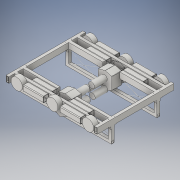
# Autodesk Inventor part: BaseSuperstructure
Saved by Autodesk Inventor 2016 (Build 200138000, 138)
## iProperties
Created: 2018-01-19
Part Number: BaseSuperstructure
Material: Generic
Document SubType Name: Modeling
Designer: New User
Density: 1 g/cm^3
Appearance: Polycarbonate - Clear
Author: New User
Autodesk Inventor part; units mm, degrees
ref_plane "YZ Plane" through (0, 0, 0) normal (1, 0, 0) x (0, 1, 0)
ref_plane "XZ Plane" through (0, 0, 0) normal (0, 1, 0) x (-1, 0, 0)
ref_plane "XY Plane" through (0, 0, 0) normal (0, 0, 1) x (1, 0, 0)
sketch "Sketch1" plane through (0, 0, 0) normal (0, 1, 0) x (-1, 0, 0)
  line L0 (0, -685.8) -> (0, 0)
  line L1 (25.4, -50.8) -> (689.3542, -50.8)
  line L2 (787.4, -76.2) -> (25.4, -76.2)
  line L3 (787.4, -635) -> (25.4, -635)
  line L4 (787.4, -609.6) -> (25.4, -609.6)
  line L5 (787.4, -127) -> (482.6, -127)
  line L6 (482.6, -127) -> (482.6, -152.4)
  line L7 (482.6, -533.4) -> (482.6, -558.8)
  line L8 (482.6, -558.8) -> (787.4, -558.8)
  line L9 (25.4, -558.8) -> (330.2, -558.8)
  line L10 (330.2, -558.8) -> (330.2, -533.4)
  line L11 (330.2, -533.4) -> (25.4, -533.4)
  line L12 (25.4, -152.4) -> (330.2, -152.4)
  line L13 (330.2, -127) -> (25.4, -127)
  line L14 (330.2, -127) -> (330.2, -152.4)
  line L15 (0, 0) -> (25.4, 0)
  line L16 (787.4, 0) -> (812.8, 0)
  line L17 (787.4, -76.2) -> (787.4, -127)
  line L18 (787.4, -558.8) -> (787.4, -609.6)
  line L19 (787.4, -635) -> (787.4, -685.8)
  line L20 (812.8, -685.8) -> (787.4, -685.8)
  line L21 (25.4, -685.8) -> (0, -685.8)
  line L22 (25.4, -635) -> (25.4, -685.8)
  line L23 (25.4, -558.8) -> (25.4, -609.6)
  line L24 (25.4, -152.4) -> (25.4, -533.4)
  line L25 (25.4, 0) -> (25.4, -50.8)
  line L26 (25.4, -76.2) -> (25.4, -127)
  line L27 (689.3542, -50.8) -> (787.4, -50.8)
  line L28 (787.4, -50.8) -> (787.4, 0)
  line L29 (812.8, 0) -> (812.8, -152.4)
  line L30 (812.8, -539.9129) -> (812.8, -685.8)
  line L31 (482.6, -152.4) -> (482.6, -152.4)
  line L32 (508, -152.4) -> (787.3559, -152.4)
  line L33 (660.3559, -533.4) -> (508, -533.4)
  line L34 (482.6, -533.4) -> (482.6, -533.4)
  line L35 (660.3559, -533.4) -> (787.3559, -533.4)
  line L36 (787.3559, -152.4) -> (787.4, -152.4)
  line L37 (787.3559, -533.4) -> (787.4, -533.4)
  line L38 (482.6, -152.4) -> (508, -152.4)
  line L39 (482.6, -533.4) -> (508, -533.4)
  line L40 (787.3559, -152.4) -> (787.3559, -533.4)
  line L41 (812.8, -539.9129) -> (812.8, -152.4)
  dimension "d0" = 685.8
  dimension "d1" = 812.8
  dimension "d4" = 25.4
  dimension "d5" = 25.4
  dimension "d8" = 50.8
  dimension "d9" = 25.4
  dimension "d10" = 50.8
  dimension "d42" = 304.8
  dimension "d43" = 25.4
  dimension "d44" = 25.4
  dimension "d45" = 25.4
  dimension "d46" = 25.4
  dimension "d101" = 50.8
  dimension "d102" = 50.8
  dimension "d103" = 25.4
  dimension "d104" = 50.8
  dimension "d105" = 25.4
  dimension "d108" = 50.8
  dimension "d117" = 50.8
  dimension "d134" = 304.8
  dimension "d135" = 304.8
  dimension "d136" = 25.4
  dimension "d137" = 25.4
  constraints: 84 end point, 63 perpendicular, 8 horizontal, 8 parallel, 6 point on line, 3 equal length
  measures "d0" distance of L16.end L20.start
  measures "d1" distance of L20.start L0.start
  measures "d4" distance between parallel lines of L3 L4
  measures "d5" distance between parallel lines of L2 L1
  measures "d8" distance between parallel lines of L4 L9
  measures "d9" distance of L9.end L10.end
  measures "d10" distance between parallel lines of L2 L5
  measures "d42" distance between parallel lines of L10 L23
  measures "d43" distance between parallel lines of L23 L0
  measures "d44" distance between parallel lines of L0 L24
  measures "d45" distance between parallel lines of L0 L26
  measures "d46" distance between parallel lines of L0 L25
  measures "d101" distance of L15.end L1.start
  measures "d102" distance between parallel lines of L2 L13
  measures "d103" distance between parallel lines of L5 L32
  measures "d104" distance of L3.start L19.end
  measures "d105" distance between parallel lines of L33 L8
  measures "d108" distance of L3.end L21.start
  measures "d117" distance of L27.end L16.start
  measures "d134" distance of L7.end L8.end
  measures "d135" distance of L5.start L5.end
  measures "d136" distance between parallel lines of L29 L17
  measures "d137" distance between parallel lines of L30 L18
extrude "Frame" add sketch "Sketch1" along normal blind 50.8
sketch "Sketch4" plane through (-25.4, 0, -76.2) normal (-1, 0, 0) x (0, 0, 1)
  line L0 (-50.8, 50.8) -> (0, 50.8) projected
  line L1 (0, 0) -> (-50.8, 0) projected
  line L2 (-6.35, 50.8) -> (-44.45, 50.8)
  line L3 (-50.8, 44.45) -> (-50.8, 6.35)
  line L4 (-44.45, 0) -> (-6.35, 0)
  line L5 (0, 6.35) -> (0, 44.45)
  arc A0 (-44.45, 50.8) -> (-50.8, 44.45) centre (-44.45, 44.45) ccw
  arc A1 (-50.8, 6.35) -> (-44.45, 0) centre (-44.45, 6.35) ccw
  arc A2 (0, 44.45) -> (-6.35, 50.8) centre (-6.35, 44.45) ccw
  arc A3 (-6.35, 0) -> (0, 6.35) centre (-6.35, 6.35) ccw
  line L6 (-533.4, 50.8) -> (-482.6, 50.8) projected
  line L7 (-482.6, 0) -> (-482.6, 50.8) projected
  line L8 (-527.05, 50.8) -> (-488.95, 50.8)
  line L9 (-482.6, 44.45) -> (-482.6, 6.35)
  line L10 (-488.95, 0) -> (-527.05, 0)
  line L11 (-533.4, 6.35) -> (-533.4, 44.45)
  arc A4 (-482.6, 44.45) -> (-488.95, 50.8) centre (-488.95, 44.45) ccw
  arc A5 (-533.4, 6.35) -> (-527.05, 0) centre (-527.05, 6.35) ccw
  arc A6 (-527.05, 50.8) -> (-533.4, 44.45) centre (-527.05, 44.45) ccw
  arc A7 (-488.95, 0) -> (-482.6, 6.35) centre (-488.95, 6.35) ccw
  line L12 (-527.05, 3.175) -> (-488.95, 3.175)
  arc A8 (-488.95, 3.175) -> (-485.775, 6.35) centre (-488.95, 6.35) ccw
  line L13 (-485.775, 6.35) -> (-485.775, 44.45)
  arc A9 (-485.775, 44.45) -> (-488.95, 47.625) centre (-488.95, 44.45) ccw
  line L14 (-488.95, 47.625) -> (-527.05, 47.625)
  arc A10 (-527.05, 47.625) -> (-530.225, 44.45) centre (-527.05, 44.45) ccw
  line L15 (-530.225, 44.45) -> (-530.225, 6.35)
  arc A11 (-530.225, 6.35) -> (-527.05, 3.175) centre (-527.05, 6.35) ccw
  line L16 (-6.35, 3.175) -> (-44.45, 3.175)
  arc A12 (-47.625, 6.35) -> (-44.45, 3.175) centre (-44.45, 6.35) ccw
  line L17 (-47.625, 6.35) -> (-47.625, 44.45)
  arc A13 (-44.45, 47.625) -> (-47.625, 44.45) centre (-44.45, 44.45) ccw
  line L18 (-44.45, 47.625) -> (-6.35, 47.625)
  arc A14 (-3.175, 44.45) -> (-6.35, 47.625) centre (-6.35, 44.45) ccw
  line L19 (-3.175, 44.45) -> (-3.175, 6.35)
  arc A15 (-6.35, 3.175) -> (-3.175, 6.35) centre (-6.35, 6.35) ccw
  line L20 (76.2, 0) -> (76.2, 50.8) projected
  line L21 (31.75, 50.8) -> (69.85, 50.8)
  line L22 (76.2, 44.45) -> (76.2, 6.35)
  line L23 (69.85, 0) -> (31.75, 0)
  line L24 (25.4, 6.35) -> (25.4, 44.45)
  line L25 (25.4, 50.8) -> (76.2, 0) construction
  line L26 (76.2, 50.8) -> (25.4, 0) construction
  arc A16 (69.85, 0) -> (76.2, 6.35) centre (69.85, 6.35) ccw
  arc A17 (76.2, 44.45) -> (69.85, 50.8) centre (69.85, 44.45) ccw
  arc A18 (31.75, 50.8) -> (25.4, 44.45) centre (31.75, 44.45) ccw
  arc A19 (25.4, 6.35) -> (31.75, 0) centre (31.75, 6.35) ccw
  line L27 (-565.15, 50.8) -> (-603.25, 50.8)
  line L28 (-609.6, 44.45) -> (-609.6, 6.35)
  line L29 (-603.25, 0) -> (-565.15, 0)
  line L30 (-558.8, 6.35) -> (-558.8, 44.45)
  line L31 (-558.8, 50.8) -> (-609.6, 0) construction
  line L32 (-609.6, 50.8) -> (-558.8, 0) construction
  arc A20 (-565.15, 0) -> (-558.8, 6.35) centre (-565.15, 6.35) ccw
  arc A21 (-558.8, 44.45) -> (-565.15, 50.8) centre (-565.15, 44.45) ccw
  arc A22 (-603.25, 50.8) -> (-609.6, 44.45) centre (-603.25, 44.45) ccw
  arc A23 (-609.6, 6.35) -> (-603.25, 0) centre (-603.25, 6.35) ccw
  line L33 (-565.15, 3.175) -> (-603.25, 3.175)
  arc A24 (-606.425, 6.35) -> (-603.25, 3.175) centre (-603.25, 6.35) ccw
  line L34 (-606.425, 6.35) -> (-606.425, 44.45)
  arc A25 (-603.25, 47.625) -> (-606.425, 44.45) centre (-603.25, 44.45) ccw
  line L35 (-603.25, 47.625) -> (-565.15, 47.625)
  arc A26 (-561.975, 44.45) -> (-565.15, 47.625) centre (-565.15, 44.45) ccw
  line L36 (-561.975, 44.45) -> (-561.975, 6.35)
  arc A27 (-565.15, 3.175) -> (-561.975, 6.35) centre (-565.15, 6.35) ccw
  line L37 (73.025, 6.35) -> (73.025, 44.45)
  arc A28 (73.025, 44.45) -> (69.85, 47.625) centre (69.85, 44.45) ccw
  line L38 (69.85, 47.625) -> (31.75, 47.625)
  arc A29 (31.75, 47.625) -> (28.575, 44.45) centre (31.75, 44.45) ccw
  line L39 (28.575, 44.45) -> (28.575, 6.35)
  arc A30 (28.575, 6.35) -> (31.75, 3.175) centre (31.75, 6.35) ccw
  line L40 (31.75, 3.175) -> (69.85, 3.175)
  arc A31 (69.85, 3.175) -> (73.025, 6.35) centre (69.85, 6.35) ccw
  point P0 (50.8, 25.4)
  point P1 (-584.2, 25.4)
  dimension "d24" = 6.35
  dimension "d25" = 6.35
  dimension "d106" = 6.35
  dimension "d109" = 6.35
  constraints: 72 end point, 64 point on circle, 32 centre point, 32 tangent, 24 point on line, 16 parallel, 12 equal radius, 8 perpendicular, 4 horizontal, 4 midpoint, 28 other
  measures "d24" radius of A0
  measures "d25" radius of A4
  measures "d106" radius of A16
  measures "d109" radius of A20
extrude "tubes" add sketch "Sketch4" along normal blind 774.7 contours L0 A2 L5 A3 L1 A1 L3 A0 | L6 A4 L7 A7 L10 A5 L11 A6 | A16 L23 A19 L24 A18 L21 A17 L20 | A21 L30 A20 L29 A23 L28 A22 L27
sketch "Sketch17" plane through (0, 0, 0) normal (0, -1, 0) x (1, 0, 0)
  line L0 (-25.4, 0) -> (-152.4, 0)
  line L1 (-152.4, 0) -> (-152.4, -50.8)
  line L2 (-152.4, -50.8) -> (-25.4, -50.8)
  line L3 (-25.4, -50.8) -> (-25.4, 0)
  line L4 (-152.4, -69.6871) -> (-25.4, -69.6871)
  line L5 (-25.4, -69.6871) -> (-25.4, -127)
  line L6 (-25.4, -127) -> (-152.4, -127)
  line L7 (-152.4, -127) -> (-152.4, -69.6871)
  line L8 (-25.4, -558.8) -> (-25.4, -565.15) projected
  line L9 (-25.4, -558.8) -> (-152.4, -558.8)
  line L10 (-152.4, -558.8) -> (-152.4, -609.6)
  line L11 (-152.4, -609.6) -> (-25.4, -609.6)
  line L12 (-25.4, -609.6) -> (-25.4, -558.8)
  line L13 (-25.4, -685.8) -> (-152.4, -685.8)
  line L14 (-152.4, -685.8) -> (-152.4, -638.175)
  line L15 (-152.4, -638.175) -> (-25.4, -638.175)
  line L16 (-25.4, -638.175) -> (-25.4, -685.8)
  line L17 (-787.4, 0) -> (-787.4, -6.35) projected
  line L18 (-787.4, 0) -> (-660.4, 0)
  line L19 (-660.4, 0) -> (-660.4, -50.8)
  line L20 (-660.4, -50.8) -> (-787.4, -50.8)
  line L21 (-787.4, -50.8) -> (-787.4, 0)
  line L22 (-787.4, -76.2) -> (-660.4, -76.2)
  line L23 (-660.4, -76.2) -> (-660.4, -127)
  line L24 (-660.4, -127) -> (-787.4, -127)
  line L25 (-787.4, -127) -> (-787.4, -76.2)
  line L26 (-787.4, -558.8) -> (-787.4, -565.15) projected
  line L27 (-787.4, -558.8) -> (-660.4, -558.8)
  line L28 (-660.4, -558.8) -> (-660.4, -609.6)
  line L29 (-660.4, -609.6) -> (-787.4, -609.6)
  line L30 (-787.4, -609.6) -> (-787.4, -558.8)
  line L31 (-787.4, -635) -> (-660.4, -635)
  line L32 (-660.4, -635) -> (-660.4, -685.8)
  line L33 (-660.4, -685.8) -> (-787.4, -685.8)
  line L34 (-787.4, -685.8) -> (-787.4, -635)
  line L35 (-330.2, 0) -> (-482.6, 0)
  line L36 (-482.6, 0) -> (-482.6, -50.8)
  line L37 (-482.6, -50.8) -> (-330.2, -50.8)
  line L38 (-330.2, -50.8) -> (-330.2, 0)
  line L39 (-330.2, -76.2) -> (-482.6, -76.2)
  line L40 (-482.6, -76.2) -> (-482.6, -127)
  line L41 (-482.6, -127) -> (-330.2, -127)
  line L42 (-330.2, -127) -> (-330.2, -76.2)
  line L43 (-482.6, -558.8) -> (-330.2, -558.8)
  line L44 (-330.2, -558.8) -> (-330.2, -609.6)
  line L45 (-330.2, -609.6) -> (-482.6, -609.6)
  line L46 (-482.6, -609.6) -> (-482.6, -558.8)
  line L47 (-330.2, -635) -> (-482.6, -635)
  line L48 (-482.6, -635) -> (-482.6, -685.8)
  line L49 (-482.6, -685.8) -> (-330.2, -685.8)
  line L50 (-330.2, -685.8) -> (-330.2, -635)
  dimension "d116" = 127
  dimension "d118" = 127
  dimension "d119" = 177.8
  dimension "d120" = 177.8
  dimension "d127" = 177.8
  dimension "d128" = 177.8
  dimension "d130" = 177.8
  dimension "d131" = 177.8
  dimension "d133" = 127
  constraints: 96 end point, 24 parallel, 12 horizontal, 12 perpendicular, 7 point on line
  measures "d116" distance of L0.start L0.end
  measures "d118" distance of L17.start L18.end
  measures "d119" distance between parallel lines of L38 L1
  measures "d120" distance between parallel lines of L19 L36
  measures "d127" distance between parallel lines of L42 L7
  measures "d128" distance between parallel lines of L23 L40
  measures "d130" distance between parallel lines of L14 L50
  measures "d131" distance between parallel lines of L32 L48
  measures "d133" distance of L5.end L6.end
extrude "Extrusion19" cut sketch "Sketch17" against normal blind 50.8
sketch "Sketch19" plane through (-787.4, 50.8, -609.6) normal (0, 0, 1) x (1, 0, 0)
  line L0 (-25.4, -50.8) -> (-25.4, 0) projected
  line L1 (319.0875, -15.875) -> (381, 0)
  line L2 (381, 0) -> (441.325, -15.875)
  line L3 (441.325, -15.875) -> (441.325, -124.4763)
  line L4 (441.325, -124.4763) -> (381, -155.575)
  line L5 (381, -155.575) -> (319.0875, -124.4763)
  line L6 (319.0875, -124.4763) -> (319.0875, -15.875)
  point P0 (787.4, -50.8)
  constraints: 12 end point, 1 parallel
extrude "Extrusion20" add sketch "Sketch19" along normal blind 131.572
sketch "Sketch23" plane through (-787.4, 0, -76.2) normal (0, 0, -1) x (-1, 0, 0)
  line L0 (-319.0875, -73.6763) -> (-381, -104.775) projected
  line L1 (-381, -104.775) -> (-319.0875, -73.6763)
  line L2 (-319.0875, 34.925) -> (-319.0875, -73.6763) projected
  line L3 (-319.0875, -73.6763) -> (-319.0875, 34.925)
  line L4 (-319.0875, 34.925) -> (-381, 50.8)
  line L5 (-441.325, -73.6763) -> (-441.325, 34.925) projected
  line L6 (-441.325, 34.925) -> (-441.325, -73.6763)
  line L7 (-441.325, -73.6763) -> (-381, -104.775)
  line L8 (-441.325, 34.925) -> (-381, 50.8)
  point P0 (-787.4, 0)
  constraints: 12 end point, 2 collinear, 1 vertical
extrude "Extrusion25" add sketch "Sketch23" along normal blind 131.572
sketch "Sketch25" plane through (-787.4, 0, -207.772) normal (0, 0, -1) x (-1, 0, 0)
  circle A0 centre (-380.3805, -90.287) radius 25.4
  circle A1 centre (-337.9892, -53.4748) radius 25.4
  circle A2 centre (-374.3738, -8.7689) radius 25.4
  point P0 (-787.4, 0)
  dimension "d170" = 50.8
  dimension "d171" = 50.8
  dimension "d172" = 50.8
  constraints: 3 centre point
  measures "d170" diameter of A0
  measures "d171" diameter of A1
  measures "d172" diameter of A2
extrude "Extrusion26" add sketch "Sketch25" along normal blind 114.3
sketch "Sketch26" plane through (-787.4, 50.8, -478.028) normal (0, 0, 1) x (1, 0, 0)
  arc A0 (355.0213, -142.5259) -> (405.7206, -142.831) centre (380.3805, -141.087) ccw projected
  circle A1 centre (380.3805, -141.087) radius 25.4
  circle A2 centre (337.9892, -104.2748) radius 25.4 projected
  circle A3 centre (337.9892, -104.2748) radius 25.4
  circle A4 centre (374.3738, -59.5689) radius 25.4 projected
  circle A5 centre (374.3738, -59.5689) radius 25.4
  point P0 (787.4, -50.8)
  point P1 (347.5192, -134.6478)
  point P2 (354.3407, -128.3917)
  constraints: 3 centre point, 3 coincident, 1 other
extrude "Extrusion27" add sketch "Sketch26" along normal blind 114.3
sketch "Sketch22" plane through (-25.4, 0.8507, -638.175) normal (0, 0, -1) x (-1, 0, 0)
  circle A0 centre (63.5, 24.5493) radius 50.8
  circle A1 centre (381, 24.5493) radius 50.8
  circle A2 centre (698.5, 24.5493) radius 50.8
  line L0 (0, -0.8507) -> (0, 49.9493) projected
  line L1 (762, -0.8507) -> (762, 49.9493) projected
  point P0 (-25.4, -0.8507)
  dimension "d154" = 101.6
  dimension "d155" = 63.5
  dimension "d156" = 381
  dimension "d157" = 63.5
  constraints: 3 centre point, 2 equal radius
  measures "d154" diameter of A2
  measures "d155" distance from line of L0 A0.centre
  measures "d156" distance from line of L0 A1.centre
  measures "d157" distance from line of L1 A2.centre
extrude "Wheels" add sketch "Sketch22" along normal blind 44.45
sketch "Sketch18" plane through (-787.4, 50.8, -50.8) normal (0, 0, 1) x (1, 0, 0)
  circle A0 centre (698.5, -25.4) radius 50.8
  circle A1 centre (63.5, -25.4) radius 50.8
  circle A2 centre (381, -25.4) radius 50.8
  line L0 (762, -50.8) -> (762, 0) projected
  line L1 (127, -6.35) -> (127, -44.45) projected
  point P0 (787.4, -50.8)
  dimension "d123" = 101.6
  dimension "d124" = 63.5
  dimension "d125" = 63.5
  dimension "d126" = 381
  constraints: 3 centre point, 2 equal radius
  measures "d123" diameter of A0
  measures "d124" distance from line of L0 A0.centre
  measures "d125" distance from line of L1 A1.centre
  measures "d126" distance from line of L0 A2.centre
extrude "Wheels2" add sketch "Sketch18" along normal blind 44.45
sketch "Sketch27" plane through (-468.3125, -73.6763, -76.2) normal (-1, 0, 0) x (0, 0, 1)
  line L0 (-527.05, -50.8) -> (-488.95, -50.8)
  line L1 (-488.95, -50.8) -> (-488.95, 149.225)
  line L2 (-488.95, 149.225) -> (-527.05, 149.225)
  line L3 (-527.05, 149.225) -> (-527.05, -50.8)
  line L4 (-44.45, -14.2875) -> (-44.45, 125.4125)
  line L5 (-44.45, 125.4125) -> (-6.35, 125.4125)
  line L6 (-6.35, 125.4125) -> (-6.35, -14.2875)
  line L7 (-6.35, -14.2875) -> (-6.35, -79.375)
  line L8 (-6.35, -79.375) -> (-44.45, -79.375)
  line L9 (-44.45, -79.375) -> (-44.45, -14.2875)
  point P0 (76.2, 73.6763)
  constraints: 20 end point, 3 parallel, 3 perpendicular, 1 horizontal, 1 vertical
extrude "Extrusion29" cut sketch "Sketch27" against normal blind 127
sketch "Sketch28" plane through (-468.3125, -73.6763, -82.55) normal (0, 0, -1) x (-1, 0, 0)
  line L0 (-115.8875, 4.7625) -> (-114.0873, 11.0555)
  line L1 (-114.0873, 11.0555) -> (-107.7373, 12.643)
  line L2 (-107.7373, 12.643) -> (-103.1875, 7.9375)
  line L3 (-103.1875, 7.9375) -> (-104.9877, 1.6445)
  line L4 (-104.9877, 1.6445) -> (-111.3377, 0.057)
  line L5 (-111.3377, 0.057) -> (-115.8875, 4.7625)
  line L6 (-68.2625, -20.6375) -> (-65.0875, -15.1382)
  line L7 (-65.0875, -15.1382) -> (-58.7375, -15.1382)
  line L8 (-58.7375, -15.1382) -> (-55.5625, -20.6375)
  line L9 (-55.5625, -20.6375) -> (-58.7375, -26.1368)
  line L10 (-58.7375, -26.1368) -> (-65.0875, -26.1368)
  line L11 (-65.0875, -26.1368) -> (-68.2625, -20.6375)
  line L12 (-17.9184, 4.7625) -> (-14.7434, 10.2618)
  line L13 (-14.7434, 10.2618) -> (-8.3934, 10.2618)
  line L14 (-8.3934, 10.2618) -> (-5.2184, 4.7625)
  line L15 (-5.2184, 4.7625) -> (-8.3934, -0.7368)
  line L16 (-8.3934, -0.7368) -> (-14.7434, -0.7368)
  line L17 (-14.7434, -0.7368) -> (-17.9184, 4.7625)
  line L18 (-105.9066, 95.25) -> (-111.9358, 92.4597)
  line L19 (-111.9358, 92.4597) -> (-117.3669, 96.2859)
  line L20 (-117.3669, 96.2859) -> (-116.7688, 102.9025)
  line L21 (-116.7688, 102.9025) -> (-110.7396, 105.6928)
  line L22 (-110.7396, 105.6928) -> (-105.3085, 101.8666)
  line L23 (-105.3085, 101.8666) -> (-105.9066, 95.25)
  line L24 (-17.9184, 98.5583) -> (-14.5168, 104.4501)
  line L25 (-14.5168, 104.4501) -> (-7.7135, 104.4501)
  line L26 (-7.7135, 104.4501) -> (-4.3119, 98.5583)
  line L27 (-4.3119, 98.5583) -> (-7.7135, 92.6665)
  line L28 (-7.7135, 92.6665) -> (-14.5168, 92.6665)
  line L29 (-14.5168, 92.6665) -> (-17.9184, 98.5583)
  point P0 (-468.3125, 73.6763)
  point P1 (-109.5375, 6.35)
  point P2 (-61.9125, -20.6375)
  point P3 (-11.5684, 4.7625)
  point P4 (-111.3377, 99.0763)
  point P5 (-11.1151, 98.5583)
  constraints: 60 end point, 65 other
extrude "Extrusion30" add sketch "Sketch28" along normal blind 65.0875
sketch "Sketch29" plane through (-468.3125, -73.6763, -565.15) normal (0, 0, -1) x (-1, 0, 0)
  line L0 (-68.2625, -20.6375) -> (-65.0875, -15.1382)
  line L1 (-65.0875, -15.1382) -> (-58.7375, -15.1382)
  line L2 (-58.7375, -15.1382) -> (-55.5625, -20.6375)
  line L3 (-55.5625, -20.6375) -> (-58.7375, -26.1368)
  line L4 (-58.7375, -26.1368) -> (-65.0875, -26.1368)
  line L5 (-65.0875, -26.1368) -> (-68.2625, -20.6375)
  line L6 (-111.125, 0) -> (-116.2712, 4.8042)
  line L7 (-116.2712, 4.8042) -> (-114.6837, 11.663)
  line L8 (-114.6837, 11.663) -> (-107.95, 13.7176)
  line L9 (-107.95, 13.7176) -> (-102.8038, 8.9134)
  line L10 (-102.8038, 8.9134) -> (-104.3913, 2.0546)
  line L11 (-104.3913, 2.0546) -> (-111.125, 0)
  line L12 (-112.7125, 106.3625) -> (-109.6472, 110.092)
  line L13 (-109.6472, 110.092) -> (-104.8847, 109.3022)
  line L14 (-104.8847, 109.3022) -> (-103.1875, 104.7828)
  line L15 (-103.1875, 104.7828) -> (-106.2528, 101.0533)
  line L16 (-106.2528, 101.0533) -> (-111.0153, 101.8431)
  line L17 (-111.0153, 101.8431) -> (-112.7125, 106.3625)
  line L18 (-16.2587, 2.0546) -> (-16.2587, 8.9134)
  line L19 (-16.2587, 8.9134) -> (-10.3188, 12.3428)
  line L20 (-10.3188, 12.3428) -> (-4.3788, 8.9134)
  line L21 (-4.3788, 8.9134) -> (-4.3788, 2.0546)
  line L22 (-4.3788, 2.0546) -> (-10.3188, -1.3748)
  line L23 (-10.3188, -1.3748) -> (-16.2587, 2.0546)
  arc A0 (-17.9184, 73.6763) -> (-17.9184, 124.4763) centre (-61.9125, 99.0763) ccw projected
  line L24 (-7.7135, 93.1867) -> (-14.0662, 92.9266)
  line L25 (-14.0662, 92.9266) -> (-17.4679, 98.2982)
  line L26 (-17.4679, 98.2982) -> (-14.5168, 103.9299)
  line L27 (-14.5168, 103.9299) -> (-8.164, 104.19)
  line L28 (-8.164, 104.19) -> (-4.7624, 98.8184)
  line L29 (-4.7624, 98.8184) -> (-7.7135, 93.1867)
  point P0 (-468.3125, 73.6763)
  point P1 (-61.9125, -20.6375)
  point P2 (-109.5375, 6.8588)
  point P3 (-107.95, 105.5727)
  point P4 (-10.3188, 5.484)
  point P5 (-11.1151, 98.5583)
  constraints: 60 end point, 1 point on circle, 1 point on line, 65 other
extrude "Extrusion31" add sketch "Sketch29" along normal blind 41.275
fillet "Fillet1" radius 3.175 11 edges at (-346.075, 34.925, -521.589) (-406.4, 50.8, -521.589) (-468.3125, 34.925, -521.589) (-468.3125, 34.925, -164.211) (-346.075, 34.925, -164.211) (-346.075, -73.6763, -164.211) (-406.4, -104.775, -164.211) (-468.3125, -73.6763, -164.211) (-406.4, -104.775, -521.589) (-346.075, -73.6763, -521.589) (-468.3125, -73.6763, -521.589)
sketch "Sketch30" plane through (0, 0, -685.8) normal (0, 0, -1) x (-1, 0, 0)
  line L0 (809.625, 3.175) -> (790.575, 3.175)
  line L1 (790.575, 3.175) -> (790.575, 47.625)
  line L2 (790.575, 47.625) -> (809.625, 47.625)
  line L3 (809.625, 47.625) -> (809.625, 3.175)
  line L4 (812.8, 0) -> (812.8, 50.8) projected
  line L5 (787.4, 0) -> (812.8, 0) projected
  line L6 (787.4, 0) -> (787.4, 50.8) projected
  line L7 (787.4, 50.8) -> (812.8, 50.8) projected
  line L8 (22.225, 3.175) -> (3.175, 3.175)
  line L9 (3.175, 3.175) -> (3.175, 47.625)
  line L10 (3.175, 47.625) -> (22.225, 47.625)
  line L11 (22.225, 47.625) -> (22.225, 3.175)
  line L12 (0, 0) -> (0, 50.8) projected
  dimension "d189" = 3.175
  dimension "d190" = 3.175
  dimension "d191" = 3.175
  dimension "d192" = 3.175
  constraints: 16 end point, 4 parallel, 2 horizontal, 2 perpendicular
  measures "d189" distance between parallel lines of L4 L3
  measures "d190" distance between parallel lines of L5 L0
  measures "d191" distance between parallel lines of L6 L1
  measures "d192" distance between parallel lines of L7 L2
extrude "Extrusion32" cut sketch "Sketch30" against normal blind 685.8 contours L0 L1 L2 L3 | L8 L9 L10 L11
sketch "Sketch33" plane through (0, 0, 0) normal (0, -1, 0) x (1, 0, 0)
  line L0 (0, 0) -> (0, -685.8) projected
  line L1 (-25.4, -152.4) -> (0, -152.4)
  line L2 (0, -152.4) -> (0, -127)
  line L3 (0, -127) -> (-25.4, -127)
  line L4 (-25.4, -127) -> (-25.4, -152.4)
  line L5 (-330.2, -533.4) -> (-25.4, -533.4) projected
  line L6 (-25.4, -533.4) -> (0, -533.4)
  line L7 (0, -533.4) -> (0, -558.8)
  line L8 (0, -558.8) -> (-25.4, -558.8)
  line L9 (-25.4, -558.8) -> (-25.4, -533.4)
  line L10 (-482.6, -127) -> (-787.4, -127) projected
  line L11 (-787.4, -127) -> (-812.8, -127)
  line L12 (-812.8, -127) -> (-812.8, -152.4)
  line L13 (-812.8, -152.4) -> (-787.4, -152.4)
  line L14 (-787.4, -152.4) -> (-787.4, -127)
  line L15 (-482.6, -558.8) -> (-787.4, -558.8) projected
  line L16 (-787.4, -558.8) -> (-812.8, -558.8)
  line L17 (-812.8, -558.8) -> (-812.8, -533.4)
  line L18 (-812.8, -533.4) -> (-787.4, -533.4)
  line L19 (-787.4, -533.4) -> (-787.4, -558.8)
  point P0 (-533.4, -127)
  constraints: 32 end point, 8 parallel, 5 point on line, 4 horizontal, 4 perpendicular
extrude "Extrusion35" add sketch "Sketch33" along normal blind 114.3
sketch "Sketch34" plane through (-812.8, 0, 0) normal (-1, 0, 0) x (0, 0, 1)
  line L0 (-152.4, -114.3) -> (-127, -114.3) projected
  line L1 (-127, -114.3) -> (-152.4, -114.3)
  line L2 (-152.4, -114.3) -> (-152.4, -139.7)
  line L3 (-152.4, -139.7) -> (-127, -139.7)
  line L4 (-127, -139.7) -> (-127, -114.3)
  line L5 (-558.8, 0) -> (-558.8, -114.3) projected
  line L6 (-558.8, -114.3) -> (-533.4, -114.3)
  line L7 (-533.4, -114.3) -> (-533.4, -139.7)
  line L8 (-533.4, -139.7) -> (-558.8, -139.7)
  line L9 (-558.8, -139.7) -> (-558.8, -114.3)
  line L10 (-555.625, -136.525) -> (-536.575, -136.525)
  line L11 (-536.575, -136.525) -> (-536.575, -117.475)
  line L12 (-536.575, -117.475) -> (-555.625, -117.475)
  line L13 (-555.625, -117.475) -> (-555.625, -136.525)
  line L14 (-130.175, -136.525) -> (-149.225, -136.525)
  line L15 (-149.225, -136.525) -> (-149.225, -117.475)
  line L16 (-149.225, -117.475) -> (-130.175, -117.475)
  line L17 (-130.175, -117.475) -> (-130.175, -136.525)
  point P0 (0, 0)
  constraints: 32 end point, 8 parallel, 4 perpendicular, 2 horizontal, 1 point on line, 6 other
extrude "Extrusion36" add sketch "Sketch34" against normal blind 812.8
sketch "Sketch35" plane through (-812.8, 0, 0) normal (-1, 0, 0) x (0, 0, 1)
  line L0 (-127, 0) -> (-101.6, 0)
  line L1 (-101.6, 0) -> (-101.6, -3.175)
  line L2 (-101.6, -3.175) -> (-123.825, -3.175)
  line L3 (-123.825, -3.175) -> (-123.825, -25.4)
  line L4 (-123.825, -25.4) -> (-127, -25.4)
  line L5 (-127, -25.4) -> (-127, 0)
  line L6 (-152.4, -25.4) -> (-152.4, 0)
  line L7 (-152.4, 0) -> (-177.8, 0)
  line L8 (-177.8, -3.175) -> (-177.8, 0)
  line L9 (-177.8, -3.175) -> (-155.575, -3.175)
  line L10 (-155.575, -3.175) -> (-155.575, -25.4)
  line L11 (-155.575, -25.4) -> (-152.4, -25.4)
  line L12 (-558.8, 0) -> (-558.8, -25.4)
  line L13 (-558.8, -25.4) -> (-561.975, -25.4)
  line L14 (-561.975, -25.4) -> (-561.975, -3.175)
  line L15 (-558.8, 0) -> (-584.2, 0)
  line L16 (-584.2, -3.175) -> (-561.975, -3.175)
  line L17 (-533.4, -25.4) -> (-533.4, 0)
  line L18 (-533.4, 0) -> (-508, 0)
  line L19 (-508, -3.175) -> (-530.225, -3.175)
  line L20 (-508, 0) -> (-508, -3.175)
  line L21 (-530.225, -3.175) -> (-530.225, -25.4)
  line L22 (-530.225, -25.4) -> (-533.4, -25.4)
  line L23 (-584.2, 0) -> (-584.2, -3.175)
  dimension "d245" = 25.4
  dimension "d246" = 25.4
  dimension "d247" = 3.175
  dimension "d248" = 3.175
  dimension "d249" = 3.175
  dimension "d250" = 3.175
  constraints: 48 end point, 8 perpendicular, 5 vertical, 3 point on line, 2 horizontal
  measures "d245" distance of L4.end L0.start
  measures "d246" distance of L0.start L0.end
  measures "d247" distance of L10.end L6.start
  measures "d248" distance of L8.start L7.end
  measures "d249" distance of L0.end L1.end
  measures "d250" distance of L3.end L4.end
extrude "Extrusion37" add sketch "Sketch35" against normal blind 25.4
sketch "Sketch37" plane through (0, 0, -685.8) normal (1, 0, 0) x (0, 0, -1)
  line L0 (-558.8, 0) -> (-558.8, -25.4)
  line L1 (-584.2, 0) -> (-584.2, -3.175) projected
  line L2 (-558.8, 0) -> (-584.2, 0)
  line L3 (-584.2, 0) -> (-584.2, -3.175)
  line L4 (-584.2, -3.175) -> (-561.975, -3.175) projected
  line L5 (-584.2, -3.175) -> (-561.975, -3.175)
  line L6 (-561.975, -3.175) -> (-561.975, -25.4) projected
  line L7 (-561.975, -3.175) -> (-561.975, -25.4)
  line L8 (-561.975, -25.4) -> (-558.8, -25.4)
  line L9 (-533.4, -25.4) -> (-533.4, 0)
  line L10 (-533.4, 0) -> (-508, 0)
  line L11 (-508, -3.175) -> (-530.225, -3.175)
  line L12 (-530.225, -3.175) -> (-530.225, -25.4)
  line L13 (-530.225, -25.4) -> (-533.4, -25.4)
  line L14 (-508, 0) -> (-508, -3.175)
  line L15 (-120.65, 0) -> (-127, 0) projected
  line L16 (-127, 0) -> (-101.6, 0)
  line L17 (-123.825, -3.175) -> (-101.6, -3.175) projected
  line L18 (-101.6, -3.175) -> (-123.825, -3.175)
  line L19 (-123.825, -3.175) -> (-123.825, -25.4)
  line L20 (-123.825, -25.4) -> (-127, -25.4)
  line L21 (-127, -25.4) -> (-127, 0)
  line L22 (-152.4, 0) -> (-152.4, -25.4)
  line L23 (-155.575, -25.4) -> (-155.575, -3.175)
  line L24 (-177.8, -3.175) -> (-155.575, -3.175) projected
  line L25 (-155.575, -3.175) -> (-177.8, -3.175)
  line L26 (-177.8, -3.175) -> (-177.8, 0)
  line L27 (-152.4, 0) -> (-177.8, 0)
  line L28 (-101.6, -3.175) -> (-101.6, 0) projected
  line L29 (-101.6, -3.175) -> (-101.6, 0)
  line L30 (-155.575, -3.175) -> (-155.575, -25.4) projected
  line L31 (-152.4, -25.4) -> (-155.575, -25.4)
  point P0 (-685.8, 0)
  constraints: 48 end point, 12 perpendicular, 6 point on line, 3 horizontal, 2 collinear, 2 vertical, 1 parallel
extrude "Extrusion38" add sketch "Sketch37" against normal blind 25.4
sketch "Sketch38" plane through (0, -25.4, -123.825) normal (0, 0, 1) x (1, 0, 0)
  circle A0 centre (-12.7, 11.1125) radius 1.5875
  circle A1 centre (-800.1, 11.1125) radius 1.5875
  point P0 (0, 25.4)
  constraints: 2 centre point
extrude "Extrusion39" cut sketch "Sketch38" against normal blind 465.1375
sketch "Sketch39" plane through (0, -3.175, -123.825) normal (0, -1, 0) x (1, 0, 0)
  circle A0 centre (-12.7, 11.1125) radius 1.5875
  circle A1 centre (-12.7, -42.8625) radius 1.5875
  circle A2 centre (-800.1, 12.7) radius 1.5875
  circle A3 centre (-800.1, -42.8625) radius 1.5875
  circle A4 centre (-800.1, -395.2875) radius 1.5875
  circle A5 centre (-800.1, -447.675) radius 1.5875
  circle A6 centre (-12.7, -395.2875) radius 1.5875
  circle A7 centre (-12.7, -449.2625) radius 1.5875
  point P0 (0, 123.825)
  constraints: 8 centre point
extrude "Extrusion40" cut sketch "Sketch39" against normal blind 69.85
fillet "Fillet2" radius 3.175 32 edges at (-25.4, -1.5875, -177.8) (0, -1.5875, -177.8) (0, -25.4, -153.9875) (-25.4, -25.4, -153.9875) (0, -25.4, -560.3875) (-25.4, -25.4, -560.3875) (-25.4, -1.5875, -584.2) (0, -1.5875, -584.2) (-25.4, -25.4, -531.8125) (0, -25.4, -531.8125) (0, -1.5875, -508) (-25.4, -1.5875, -508) (-25.4, -25.4, -125.4125) (0, -25.4, -125.4125) (0, -1.5875, -101.6) (-25.4, -1.5875, -101.6) (-787.4, -25.4, -125.4125) (-812.8, -25.4, -125.4125) (-787.4, -1.5875, -101.6) (-812.8, -1.5875, -101.6) (-787.4, -25.4, -531.8125) (-812.8, -25.4, -531.8125) (-787.4, -1.5875, -508) (-812.8, -1.5875, -508) (-787.4, -25.4, -153.9875) (-812.8, -25.4, -153.9875) (-812.8, -1.5875, -177.8) (-787.4, -1.5875, -177.8) (-787.4, -25.4, -560.3875) (-812.8, -25.4, -560.3875) (-812.8, -1.5875, -584.2) (-787.4, -1.5875, -584.2)
sketch "Sketch40" plane through (-330.2, 50.8, -533.4) normal (0, 0, 1) x (1, 0, 0)
  line L0 (-457.2, -165.1) -> (304.8, -165.1) projected
  line L1 (304.8, -165.1) -> (26.9875, -53.975)
  line L2 (26.9875, -53.975) -> (27.6444, -52.3328)
  line L3 (27.6444, -52.3328) -> (305.4569, -163.4578)
  line L4 (305.4569, -163.4578) -> (304.8, -165.1)
  point P0 (330.2, -50.8)
  constraints: 8 end point, 2 parallel, 1 perpendicular
revolve "Revolution1" add sketch "Sketch40" angle 360 about axis through (-302.5556, -1.5328, -533.4) along (0.9284767, -0.3713907, 0)
sketch "Sketch41" plane through (-787.3559, 0, -533.4) normal (0, 0, 1) x (1, 0, 0)
  line L0 (269.8309, -3.175) -> (285.7059, -3.175) projected
  line L1 (0, -114.3) -> (277.7684, -3.175)
  line L2 (277.7684, -3.175) -> (277.3364, -2.0953)
  line L3 (277.3364, -2.0953) -> (-0.432, -113.2203)
  line L4 (-0.432, -113.2203) -> (0, -114.3)
  point P0 (787.3559, 0)
  constraints: 8 end point, 2 parallel, 1 midpoint, 1 perpendicular
revolve "Revolution2" add sketch "Sketch41" angle 360 about axis through (-510.0195, -2.0953, -533.4) along (-0.9284564, -0.3714415, 0)
sketch "Sketch42" plane through (-787.3559, 0, -533.4) normal (0, 0, 1) x (1, 0, 0)
  line L0 (-0.0441, 0) -> (-0.0441, 50.8) projected
  line L1 (-0.0441, -114.3) -> (761.9559, -114.3) projected
  line L2 (-0.0441, 0) -> (277.7684, -114.3)
  line L3 (277.7684, -114.3) -> (278.1355, -113.4078)
  line L4 (278.1355, -113.4078) -> (0.323, 0.8922)
  line L5 (0.323, 0.8922) -> (-0.0441, 0)
  point P0 (787.3559, 0)
  point P1 (0, 0)
  dimension "d266" = 0.3671
  constraints: 8 end point, 2 parallel, 1 perpendicular, 1 point on line
  measures "d266" horizontal distance of L2.end L3.end
revolve "Revolution3" add sketch "Sketch42" angle 360 about axis through (-787.4, 0, -533.4) along (0.9247875, -0.380484, 0)
sketch "Sketch43" plane through (-330.2, 50.8, -533.4) normal (0, 0, 1) x (1, 0, 0)
  line L0 (304.8, -50.8) -> (304.8, 0) projected
  line L1 (-179.3875, -165.1) -> (304.8, -165.1) projected
  line L2 (304.8, -50.8) -> (23.8125, -165.1)
  line L3 (23.8125, -165.1) -> (23.3617, -163.9918)
  line L4 (23.3617, -163.9918) -> (304.3492, -49.6918)
  line L5 (304.3492, -49.6918) -> (304.8, -50.8)
  point P0 (330.2, -50.8)
  constraints: 8 end point, 2 parallel, 1 perpendicular, 1 point on line
revolve "Revolution4" add sketch "Sketch43" angle 360 about axis through (-306.8383, -113.1918, -533.4) along (0.9262954, 0.3767981, 0)
sketch "Sketch44" plane through (-25.4, 50.8, -152.4) normal (0, 0, -1) x (-1, 0, 0)
  line L0 (0, -50.8) -> (762, -50.8) projected
  line L1 (0, -50.8) -> (280.9875, -165.1)
  line L2 (280.9875, -165.1) -> (281.4383, -163.9918)
  line L3 (281.4383, -163.9918) -> (0.4508, -49.6918)
  line L4 (0.4508, -49.6918) -> (0, -50.8)
  line L5 (0, -50.8) -> (136.9519, -106.5092) projected
  point P0 (281.8891, -162.8837)
  point P1 (260.35, -50.8)
  constraints: 8 end point, 2 parallel, 1 collinear, 1 perpendicular
revolve "Revolution5" add sketch "Sketch44" angle 360 about axis through (-306.8383, -113.1918, -152.4) along (0.9262954, 0.3767981, 0)
sketch "Sketch46" plane through (-25.4, 50.8, -152.4) normal (0, 0, -1) x (-1, 0, 0)
  line L0 (271.4625, -53.975) -> (287.3375, -53.975) projected
  line L1 (0, -73.025) -> (0, -165.1) projected
  line L2 (277.8125, -53.975) -> (0, -165.1)
  line L3 (0, -165.1) -> (-0.6569, -163.4578)
  line L4 (-0.6569, -163.4578) -> (277.1556, -52.3328)
  line L5 (277.1556, -52.3328) -> (277.8125, -53.975)
  point P0 (-25.4, -50.8)
  constraints: 8 end point, 2 parallel, 1 perpendicular, 1 point on line
revolve "Revolution6" add sketch "Sketch46" angle 360 about axis through (-24.7431, -112.6578, -152.4) along (-0.9284767, 0.3713907, 0)
sketch "Sketch47" plane through (0, -139.7, -152.4) normal (0, 0, -1) x (-1, 0, 0)
  line L0 (787.4, 25.4) -> (509.5875, 136.525)
  line L1 (509.5875, 136.525) -> (510.0194, 137.6048)
  line L2 (510.0194, 137.6048) -> (787.8319, 26.4798)
  line L3 (787.8319, 26.4798) -> (787.4, 25.4)
  point P0 (0, 139.7)
  constraints: 8 end point, 2 parallel, 1 perpendicular
revolve "Revolution7" add sketch "Sketch47" angle 360 about axis through (-510.0194, -2.0952, -152.4) along (-0.9284767, -0.3713907, 0)
sketch "Sketch48" plane through (0, -139.7, -152.4) normal (0, 0, -1) x (-1, 0, 0)
  line L0 (787.4, 138.6568) -> (650.8992, 82.4965) projected
  line L1 (509.9546, 24.5078) -> (512.1231, 25.4) projected
  line L2 (787.4, 138.6568) -> (509.9546, 24.5078)
  line L3 (509.9546, 24.5078) -> (509.5875, 25.4)
  line L4 (509.5875, 25.4) -> (787.0329, 139.549)
  line L5 (787.0329, 139.549) -> (787.4, 138.6568)
  point P0 (0, 139.7)
  constraints: 8 end point, 2 parallel, 1 collinear, 1 perpendicular, 1 point on line
revolve "Revolution8" add sketch "Sketch48" angle 360 about axis through (-509.5875, -114.3, -152.4) along (-0.9247875, 0.380484, 0)
sketch "Sketch32" plane through (0, 0, 0) normal (0, -1, 0) x (1, 0, 0)
  line L0 (-323.85, -152.4) -> (-285.75, -152.4)
  line L1 (-279.4, -146.05) -> (-279.4, -57.15)
  line L2 (-285.75, -50.8) -> (-323.85, -50.8)
  line L3 (-330.2, -57.15) -> (-330.2, -146.05)
  arc A0 (-330.2, -146.05) -> (-323.85, -152.4) centre (-323.85, -146.05) ccw
  arc A1 (-285.75, -152.4) -> (-279.4, -146.05) centre (-285.75, -146.05) ccw
  arc A2 (-279.4, -57.15) -> (-285.75, -50.8) centre (-285.75, -57.15) ccw
  arc A3 (-323.85, -50.8) -> (-330.2, -57.15) centre (-323.85, -57.15) ccw
  line L4 (-330.2, -533.4) -> (-330.2, -558.8) projected
  line L5 (-323.85, -533.4) -> (-285.75, -533.4)
  line L6 (-279.4, -539.75) -> (-279.4, -628.65)
  line L7 (-285.75, -635) -> (-323.85, -635)
  line L8 (-330.2, -628.65) -> (-330.2, -539.75)
  arc A4 (-330.2, -628.65) -> (-323.85, -635) centre (-323.85, -628.65) ccw
  arc A5 (-285.75, -635) -> (-279.4, -628.65) centre (-285.75, -628.65) ccw
  arc A6 (-279.4, -539.75) -> (-285.75, -533.4) centre (-285.75, -539.75) ccw
  arc A7 (-323.85, -533.4) -> (-330.2, -539.75) centre (-323.85, -539.75) ccw
  circle A8 centre (-317.5, -622.3) radius 1.5875
  circle A9 centre (-304.8, -622.3) radius 1.5875
  circle A10 centre (-292.1, -622.3) radius 1.5875
  circle A11 centre (-317.5, -546.1) radius 1.5875
  circle A12 centre (-304.8, -546.3264) radius 1.5875
  circle A13 centre (-292.1, -546.1) radius 1.5875
  circle A14 centre (-317.5, -139.7) radius 1.5875
  circle A15 centre (-304.8, -139.7) radius 1.5875
  circle A16 centre (-292.1, -139.7) radius 1.5875
  circle A17 centre (-317.5, -63.5) radius 1.5875
  circle A18 centre (-304.8, -63.5) radius 1.5875
  circle A19 centre (-292.1, -63.5) radius 1.5875
  line L9 (-312.7375, -127) -> (-298.45, -127)
  line L10 (-292.1, -120.65) -> (-292.1, -82.55)
  line L11 (-298.45, -76.2) -> (-312.7375, -76.2)
  line L12 (-319.0875, -82.55) -> (-319.0875, -120.65)
  arc A20 (-319.0875, -120.65) -> (-312.7375, -127) centre (-312.7375, -120.65) ccw
  arc A21 (-298.45, -127) -> (-292.1, -120.65) centre (-298.45, -120.65) ccw
  arc A22 (-292.1, -82.55) -> (-298.45, -76.2) centre (-298.45, -82.55) ccw
  arc A23 (-312.7375, -76.2) -> (-319.0875, -82.55) centre (-312.7375, -82.55) ccw
  line L13 (-312.7375, -609.6) -> (-296.8625, -609.6)
  line L14 (-290.5125, -603.25) -> (-290.5125, -565.15)
  line L15 (-296.8625, -558.8) -> (-312.7375, -558.8)
  line L16 (-319.0875, -565.15) -> (-319.0875, -603.25)
  arc A24 (-319.0875, -603.25) -> (-312.7375, -609.6) centre (-312.7375, -603.25) ccw
  arc A25 (-296.8625, -609.6) -> (-290.5125, -603.25) centre (-296.8625, -603.25) ccw
  arc A26 (-290.5125, -565.15) -> (-296.8625, -558.8) centre (-296.8625, -565.15) ccw
  arc A27 (-312.7375, -558.8) -> (-319.0875, -565.15) centre (-312.7375, -565.15) ccw
  line L17 (-488.95, -533.4) -> (-527.05, -533.4)
  line L18 (-533.4, -539.75) -> (-533.4, -628.65)
  line L19 (-527.05, -635) -> (-488.95, -635)
  line L20 (-482.6, -628.65) -> (-482.6, -539.75)
  arc A28 (-533.4, -628.65) -> (-527.05, -635) centre (-527.05, -628.65) ccw
  arc A29 (-488.95, -635) -> (-482.6, -628.65) centre (-488.95, -628.65) ccw
  arc A30 (-482.6, -539.75) -> (-488.95, -533.4) centre (-488.95, -539.75) ccw
  arc A31 (-527.05, -533.4) -> (-533.4, -539.75) centre (-527.05, -539.75) ccw
  line L21 (-488.95, -152.4) -> (-527.05, -152.4)
  line L22 (-533.4, -146.05) -> (-533.4, -57.15)
  line L23 (-527.05, -50.8) -> (-488.95, -50.8)
  line L24 (-482.6, -57.15) -> (-482.6, -146.05)
  arc A32 (-533.4, -146.05) -> (-527.05, -152.4) centre (-527.05, -146.05) ccw
  arc A33 (-488.95, -152.4) -> (-482.6, -146.05) centre (-488.95, -146.05) ccw
  arc A34 (-482.6, -57.15) -> (-488.95, -50.8) centre (-488.95, -57.15) ccw
  arc A35 (-527.05, -50.8) -> (-533.4, -57.15) centre (-527.05, -57.15) ccw
  circle A36 centre (-520.7, -139.7) radius 1.5875
  circle A37 centre (-508, -139.7) radius 1.5875
  circle A38 centre (-495.3, -139.7) radius 1.5875
  circle A39 centre (-495.3, -63.5) radius 1.5875
  circle A40 centre (-508, -63.5) radius 1.5875
  circle A41 centre (-520.7, -63.5) radius 1.5875
  circle A42 centre (-522.2875, -546.1) radius 1.5875
  circle A43 centre (-509.5875, -546.1) radius 1.5875
  circle A44 centre (-496.8875, -546.1) radius 1.5875
  circle A45 centre (-495.3, -622.3) radius 1.5875
  circle A46 centre (-508, -622.3) radius 1.5875
  circle A47 centre (-520.7, -622.3) radius 1.5875
  line L25 (-517.525, -609.6) -> (-501.65, -609.6)
  line L26 (-495.3, -603.25) -> (-495.3, -565.15)
  line L27 (-501.65, -558.8) -> (-517.525, -558.8)
  line L28 (-523.875, -565.15) -> (-523.875, -603.25)
  line L29 (-515.9375, -127) -> (-500.0625, -127)
  line L30 (-493.7125, -120.65) -> (-493.7125, -82.55)
  line L31 (-500.0625, -76.2) -> (-515.9375, -76.2)
  line L32 (-522.2875, -82.55) -> (-522.2875, -120.65)
  arc A48 (-522.2875, -120.65) -> (-515.9375, -127) centre (-515.9375, -120.65) ccw
  arc A49 (-500.0625, -127) -> (-493.7125, -120.65) centre (-500.0625, -120.65) ccw
  arc A50 (-493.7125, -82.55) -> (-500.0625, -76.2) centre (-500.0625, -82.55) ccw
  arc A51 (-515.9375, -76.2) -> (-522.2875, -82.55) centre (-515.9375, -82.55) ccw
  arc A52 (-517.525, -558.8) -> (-523.875, -565.15) centre (-517.525, -565.15) ccw
  arc A53 (-495.3, -565.15) -> (-501.65, -558.8) centre (-501.65, -565.15) ccw
  arc A54 (-501.65, -609.6) -> (-495.3, -603.25) centre (-501.65, -603.25) ccw
  arc A55 (-523.875, -603.25) -> (-517.525, -609.6) centre (-517.525, -603.25) ccw
  point P0 (0, 0)
  point P1 (-330.2, -152.4)
  point P2 (-279.4, -152.4)
  point P3 (-279.4, -635)
  point P4 (-292.1, -76.2)
  point P5 (-290.5125, -558.8)
  point P6 (-482.6, -533.4)
  point P7 (-533.4, -635)
  point P8 (-533.4, -50.8)
  point P9 (-523.875, -609.6)
  point P10 (-495.3, -558.8)
  point P11 (-522.2875, -127)
  point P12 (-493.7125, -76.2)
  dimension "d197" = 50.8
  dimension "d198" = 6.35
  dimension "d200" = 6.35
  dimension "d201" = 12.7
  dimension "d202" = 12.7
  dimension "d203" = 12.7
  dimension "d204" = 12.7
  dimension "d205" = 12.7
  dimension "d206" = 12.7
  dimension "d207" = 6.35
  dimension "d208" = 6.35
  dimension "d211" = 6.35
  dimension "d215" = 12.7
  dimension "d216" = 12.7
  dimension "d220" = 6.35
  dimension "d224" = 12.7
  dimension "d225" = 12.7
  dimension "d226" = 12.7
  dimension "d227" = 12.7
  dimension "d229" = 12.7
  dimension "d230" = 12.7
  dimension "d231" = 12.7
  dimension "d232" = 12.7
  dimension "d234" = 12.7
  dimension "d235" = 12.7
  dimension "d236" = 12.7
  dimension "d238" = 6.35
  constraints: 64 end point, 64 point on circle, 64 tangent, 56 centre point, 26 point on line, 25 equal radius, 16 parallel, 8 horizontal, 8 perpendicular
  measures "d197" distance of point (-330.2, -152.4) point (-279.4, -152.4)
  measures "d198" radius of A0
  measures "d200" radius of A4
  measures "d201" horizontal distance of A12.centre A11.centre
  measures "d202" horizontal distance of A13.centre A12.centre
  measures "d203" distance of A9.centre A8.centre
  measures "d204" distance of A10.centre A9.centre
  measures "d205" distance of A15.centre A14.centre
  measures "d206" distance of A15.centre A16.centre
  measures "d207" radius of A20
  measures "d208" radius of A24
  measures "d211" radius of A28
  measures "d215" distance from line of L3 A14.centre
  measures "d216" distance from line of L8 A11.centre
  measures "d220" radius of A32
  measures "d224" distance of A39.centre A40.centre
  measures "d225" distance of A41.centre A40.centre
  measures "d226" distance from line of L22 A41.centre
  measures "d227" distance from line of L22 A36.centre
  measures "d229" distance of A37.centre A38.centre
  measures "d230" distance from line of L21 A37.centre
  measures "d231" distance from line of L18 A47.centre
  measures "d232" distance of A47.centre A46.centre
  measures "d234" distance from line of L20 A45.centre
  measures "d235" distance of A45.centre A46.centre
  measures "d236" distance of A37.centre A36.centre
  measures "d238" radius of A48
extrude "Extrusion41" add sketch "Sketch32" along normal blind 3.175
body "Solid1"
